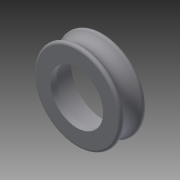
# Autodesk Inventor part: bearingPulley
Saved by Autodesk Inventor 2014 (Build 180170000, 170)
## iProperties
Created: 2013-12-16
Part Number: bearingPulley
Material: Generic
Document SubType Name: Modeling
Designer: Peele
Density: 1 g/cm^3
Appearance: Default
Author: Peele
Autodesk Inventor part; units mm, degrees
ref_plane "YZ Plane" through (0, 0, 0) normal (1, 0, 0) x (0, 1, 0)
ref_plane "XZ Plane" through (0, 0, 0) normal (0, 1, 0) x (-1, 0, 0)
ref_plane "XY Plane" through (0, 0, 0) normal (0, 0, 1) x (1, 0, 0)
sketch "Sketch1" plane through (0, 0, 0) normal (1, 0, 0) x (0, 1, 0)
  line L0 (0, 0) -> (0, 7) construction
  line L1 (11, 0) -> (11, 7)
  line L2 (11, 7) -> (9, 7)
  line L3 (9, 7) -> (9, 9)
  line L4 (9, 9) -> (14, 9)
  line L5 (11, 0) -> (14, 0)
  arc A0 (14.5851, 7.4744) -> (14, 9) centre (14, 8.125) ccw
  arc A1 (14.5851, 7.4744) -> (14.5851, 1.5256) centre (17.2596, 4.5) ccw
  arc A2 (14, 0) -> (14.5851, 1.5256) centre (14, 0.875) ccw
  line L6 (14.875, 0.875) -> (14.875, -2.7883) construction
  line L7 (13.2596, 4.5) -> (13.2596, 8) construction
  dimension "d0" = 7
  dimension "d1" = 11
  dimension "d2" = 2
  dimension "d3" = 2
  dimension "d5" = 3
  dimension "d6" = 4
  dimension "d7" = 0.875
  dimension "d9" = 13.2596
  dimension "d10" = 14.875
  constraints: 16 end point, 8 point on circle, 5 parallel, 4 tangent, 3 centre point, 3 vertical alignment, 2 horizontal alignment, 2 perpendicular, 1 equal radius, 1 vertical
  measures "d0" distance of L0.start L0.end
  measures "d1" distance between parallel lines of L0 L1
  measures "d2" distance of L1.end L2.end
  measures "d3" distance of L2.end L3.end
  measures "d5" distance from line of A0.centre L1
  measures "d6" radius of A1
  measures "d7" radius of A0
  measures "d9" distance between parallel lines of L7 L0
  measures "d10" distance between parallel lines of L0 L6
revolve "Revolution1" add sketch "Sketch1" angle 360 about axis through (0, 0, 0) along (0, 0, 1)
body "Solid1"
